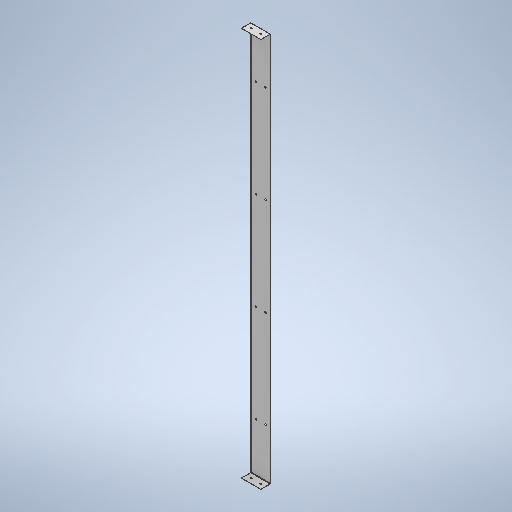
# Autodesk Inventor part: A1_BeamCoverPlate
Saved by Autodesk Inventor 2025.2 (Build 292293000, 293)
## iProperties
Created: 2025-03-18
Part Number: A1_BeamCoverPlate
Material: Generic
Document SubType Name: Sheet Metal
Designer: Victor
Density: 1 g/cm^3
Sheet Metal Rule: Default_mm
Appearance: Default
Author: Victor
Autodesk Inventor part; units mm, degrees
ref_plane "YZ Plane" through (0, 0, 0) normal (1, 0, 0) x (0, 1, 0)
ref_plane "XZ Plane" through (0, 0, 0) normal (0, 1, 0) x (-1, 0, 0)
ref_plane "XY Plane" through (0, 0, 0) normal (0, 0, 1) x (1, 0, 0)
sketch "Sketch1" plane through (0, 0, 0) normal (0, 0, 1) x (1, 0, 0)
  line L0 (0, 0) -> (50, 0)
  line L1 (50, 0) -> (50, 1000)
  line L2 (50, 1000) -> (0, 1000)
  line L3 (0, 1000) -> (0, 0)
  dimension "d0" = 50
  dimension "d1" = 1000
  measures "d0" distance of L2.end L1.end
  measures "d1" distance of L1.end L0.end
extrude "Plate1" add sketch "Sketch1" along normal blind 0.5
sketch "Sketch2" plane through (0, 0, 0.5) normal (0, 0, 1) x (1, 0, 0)
  circle A0 centre (12.5, 125) radius 2
  line L0 (50, 0) -> (0, 0) projected
  line L1 (0, 0) -> (0, 1000) projected
  circle A1 centre (12.5, 375) radius 2
  circle A2 centre (12.5, 625) radius 2
  circle A3 centre (12.5, 875) radius 2
  circle A4 centre (37.5, 875) radius 2
  line L2 (50, 1000) -> (50, 0) projected
  line L3 (0, 1000) -> (50, 1000) projected
  circle A5 centre (37.5, 625) radius 2
  circle A6 centre (37.5, 375) radius 2
  circle A7 centre (37.5, 125) radius 2
  dimension "d3" = 4
  dimension "d4" = 125
  dimension "d5" = 12.5
  dimension "d6" = 4
  dimension "d7" = 250
  dimension "d8" = 12.5
  dimension "d9" = 4
  dimension "d10" = 250
  dimension "d11" = 12.5
  dimension "d12" = 4
  dimension "d13" = 250
  dimension "d14" = 12.5
  dimension "d15" = 4
  dimension "d16" = 12.5
  dimension "d17" = 125
  dimension "d18" = 4
  dimension "d19" = 250
  dimension "d20" = 12.5
  dimension "d21" = 4
  dimension "d22" = 250
  dimension "d23" = 12.5
  dimension "d24" = 4
  dimension "d25" = 250
  dimension "d26" = 12.5
  constraints: 8 centre point
  measures "d3" diameter of A0
  measures "d4" distance from line of L0 A0.centre
  measures "d5" distance from line of L1 A0.centre
  measures "d6" diameter of A1
  measures "d7" distance of A0.centre A1.centre
  measures "d8" distance from line of L1 A1.centre
  measures "d9" diameter of A2
  measures "d10" distance of A1.centre A2.centre
  measures "d11" distance from line of L1 A2.centre
  measures "d12" diameter of A3
  measures "d13" distance of A2.centre A3.centre
  measures "d14" distance from line of L1 A3.centre
  measures "d15" diameter of A4
  measures "d16" distance from line of L2 A4.centre
  measures "d17" distance from line of L3 A4.centre
  measures "d18" diameter of A5
  measures "d19" distance of A4.centre A5.centre
  measures "d20" distance from line of L2 A5.centre
  measures "d21" diameter of A6
  measures "d22" distance of A6.centre A5.centre
  measures "d23" distance from line of L2 A6.centre
  measures "d24" diameter of A7
  measures "d25" distance of A6.centre A7.centre
  measures "d26" distance from line of L2 A7.centre
hole "Hole1" at (12.5, 875, 0.5) at (37.5, 875, 0.5) at (37.5, 625, 0.5) at (12.5, 625, 0.5) at (37.5, 375, 0.5) at (12.5, 375, 0.5) at (37.5, 125, 0.5) at (12.5, 125, 0.5) direction (0, 0, -1) diameter 4 end through all
sketch "Sketch3" plane through (0, 999.5, 0) normal (0, 1, 0) x (-1, 0, 0)
  line L0 (-50, 0) -> (0, 0)
  line L1 (0, 0) -> (0, 25)
  line L2 (0, 25) -> (-50, 25)
  line L3 (-50, 25) -> (-50, 0)
  constraints: 6 end point, 1 horizontal, 1 perpendicular, 1 vertical
edge flange "Flange1" height 25 angle 90 thickness 0.5 bend radius 0.5 thickness toward (0, 1, 0) relief straight relief width 0.5 relief depth 0.25 edges at (25, 1000, 0.5) wall of the first edge with corners at (50, 999.5, 0) (0, 999.5, 0) (0, 999.5, 25) (50, 999.5, 25)
bend "Bend1"
corner "Corner1"
sketch "Sketch4" plane through (50, 0.5, 0) normal (0, -1, 0) x (1, 0, 0)
  line L0 (-50, 0) -> (0, 0)
  line L1 (0, 0) -> (0, 25)
  line L2 (0, 25) -> (-50, 25)
  line L3 (-50, 25) -> (-50, 0)
  constraints: 6 end point, 1 horizontal, 1 perpendicular, 1 vertical
edge flange "Flange2" height 25 angle 90 thickness 0.5 bend radius 0.5 thickness toward (0, -1, 0) relief straight relief width 0.5 relief depth 0.25 edges at (25, 0, 0.5) wall of the first edge with corners at (0, 0.5, 0) (50, 0.5, 0) (50, 0.5, 25) (0, 0.5, 25)
bend "Bend2"
corner "Corner2"
sketch "Sketch5" plane through (0, 1000, 25) normal (0, 1, 0) x (1, 0, 0)
  circle A0 centre (12.5, 12.5) radius 2
  circle A1 centre (37.5, 12.5) radius 2
  line L0 (0, 0) -> (0, 24) projected
  line L1 (50, 24) -> (50, 0) projected
  line L2 (50, 0) -> (0, 0) projected
  point P0 (0, 25)
  dimension "d54" = 4
  dimension "d55" = 4
  dimension "d56" = 12.5
  dimension "d57" = 12.5
  dimension "d58" = 12.5
  dimension "d59" = 12.5
  constraints: 2 centre point
  measures "d54" diameter of A0
  measures "d55" diameter of A1
  measures "d56" distance from line of L0 A0.centre
  measures "d57" distance from line of L1 A1.centre
  measures "d58" distance from line of L2 A1.centre
  measures "d59" distance from line of L2 A0.centre
hole "Hole2" at (12.5, 1000, 12.5) at (37.5, 1000, 12.5) direction (0, -1, 0) diameter 4 end through all
equation "\"d0\" = A_width"
equation "\"d1\" = A_length"
equation "\"d3\" = rivet_diameter"
equation "\"d4\" = 0.5 * rivet_displacement"
equation "\"d5\" = 0.25 * A_width"
equation "\"d6\" = rivet_diameter"
equation "\"d7\" = rivet_displacement"
equation "\"d8\" = 0.25 * A_width"
equation "\"d9\" = rivet_diameter"
equation "\"d10\" = rivet_displacement"
equation "\"d11\" = 0.25 * A_width"
equation "\"d12\" = rivet_diameter"
equation "\"d13\" = rivet_displacement"
equation "\"d14\" = 0.25 * A_width"
equation "\"d15\" = rivet_diameter"
equation "\"d16\" = 0.25 * A_width"
equation "\"d17\" = 0.5 * rivet_displacement"
equation "\"d18\" = rivet_diameter"
equation "\"d19\" = rivet_displacement"
equation "\"d20\" = 0.25 * A_width"
equation "\"d21\" = rivet_diameter"
equation "\"d22\" = rivet_displacement"
equation "\"d23\" = 0.25 * A_width"
equation "\"d24\" = rivet_diameter"
equation "\"d25\" = rivet_displacement"
equation "\"d26\" = 0.25 * A_width"
equation "\"d27\" = rivet_diameter"
equation "\"d32\" = Thickness"
equation "\"d54\" = rivet_diameter"
equation "\"d55\" = rivet_diameter"
equation "\"d56\" = 0.25 * A_width"
equation "\"d57\" = 0.25 * A_width"
equation "\"d58\" = 0.25 * A_width"
equation "\"d59\" = 0.25 * A_width"
equation "\"d60\" = rivet_diameter"
equation "\"d65\" = Thickness"
equation "\"d2\" = Thickness"
equation "\"d34\" = BendReliefWidth"
equation "\"d35\" = BendReliefDepth"
equation "\"d36\" = MinimumRemnant"
equation "\"d37\" = TransitionRadius"
equation "\"d38\" = 0.5 * A_width"
equation "\"d40\" = BendRadius"
equation "\"d41\" = CornerReliefSize"
equation "\"d42\" = GapSize"
equation "\"d43\" = JacobiRadiusSize"
equation "\"d44\" = BendReliefWidth"
equation "\"d45\" = BendReliefDepth"
equation "\"d46\" = MinimumRemnant"
equation "\"d47\" = TransitionRadius"
equation "\"d48\" = 0.5 * A_width"
equation "\"d50\" = BendRadius"
equation "\"d51\" = CornerReliefSize"
equation "\"d52\" = GapSize"
equation "\"d53\" = JacobiRadiusSize"
equation "\"BendRadius\" = Thickness"
equation "\"BendReliefWidth\" = Thickness"
equation "\"BendReliefDepth\" = 0.5 * Thickness"
equation "\"CornerReliefSize\" = 4 * Thickness"
equation "\"MinimumRemnant\" = 2 * Thickness"
equation "\"TransitionRadius\" = BendRadius"
equation "\"JacobiRadiusSize\" = BendRadius"
equation "\"GapSize\" = Thickness"
equation "\"A_length\" = 1000"
equation "\"A_width\" = 50"
equation "\"l___________\" = 0"
equation "\"l__________\" = 0"
equation "\"l_________\" = 0"
equation "\"rivet_diameter\" = 4"
equation "\"rivet_displacement\" = 250"
equation "\"l________\" = 0"
equation "\"Thickness\" = 0.5"
body "Solid1"
